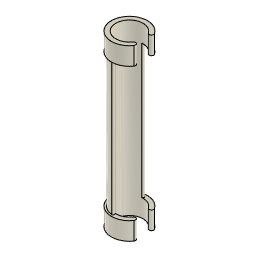
LaptopArmHolder v2 (Autodesk Fusion 360 design; units mm, degrees)
Autodesk Fusion 360 part; units mm, degrees
sketch "Sketch1" plane through (0, 0, 0) normal (0, 0, 1) x (1, 0, 0)
  circle A0 centre (14.5763, 12.4188) radius 15.25
  circle A1 centre (14.5763, 12.4188) radius 18.25
  circle A2 centre (14.5763, 12.4188) radius 20.25
  line L0 (14.5763, 32.6688) -> (14.5763, -7.8312)
  dimension "d1" = 30.5
  dimension "d2" = 36.5
  dimension "d6" = 40.5
  constraint concentric A0 A1
  constraint concentric A1 A2
  constraint coincident A2 L0.start
  constraint coincident A2 L0.end
  constraint vertical L0
  measures "d1" diameter of A0
  measures "d2" diameter of A1
  measures "d6" diameter of A2
extrude "Extrude1" add sketch "Sketch1" along normal blind 150 contours A0 A1 L0 picked at (13.6696, 29.6009)
sketch "Sketch2" plane through (0, 0, 150) normal (0, 0, 1) x (-1, 0, 0)
  arc A0 (-14.5763, -30.6688) -> (-14.5763, 5.8312) centre (-14.5763, -12.4188) ccw
  arc A1 (-14.5763, -27.6688) -> (-14.5763, 2.8312) centre (-14.5763, -12.4188) ccw
  circle A2 centre (-14.5763, -12.4188) radius 15.25
  circle A3 centre (-14.5763, -12.4188) radius 20.25
  line L0 (-14.5763, -32.6688) -> (-14.5763, 7.8312)
  line L1 (-14.5763, -27.6688) -> (-14.5763, -30.6688)
  line L2 (-14.5763, 5.8312) -> (-14.5763, 2.8312)
  line L3 (-14.5763, -27.6688) -> (-14.5763, -12.4188)
  line L4 (-14.5763, 2.8312) -> (-14.5763, -12.4188)
  line L5 (-14.5763, -4.7938) -> (-33.3359, -4.7938)
  line L6 (-14.5763, -20.0438) -> (-33.3359, -20.0438)
  dimension "d5" = 40.5
  constraint concentric A0 A2
  constraint concentric A2 A3
  constraint coincident A3 L0.start
  constraint coincident A3 L0.end
  constraint coincident A1.start L1.start
  constraint coincident A0.centre A1.centre
  constraint parallel L0 L3
  constraint coincident A1.end L2.end
  constraint midpoint L4 L5.start
  constraint coincident A3 L5.end
  constraint perpendicular L4 L5
  constraint midpoint L3 L6.start
  constraint coincident A3 L6.end
  constraint perpendicular L3 L6
  measures "d5" diameter of A3
extrude "Extrude2" add sketch "Sketch2" along normal blind 20 contours A0 A1 A2 L0 L1 L2 | A0 A3 L0 | A2 A3 L0 L1 L6 | A2 A3 L0 L2 L5
sketch "Sketch3" plane through (0, 0, 0) normal (0, 0, 1) x (1, 0, 0)
  circle A0 centre (14.5763, 12.4188) radius 15.25
  line L0 (14.5763, 32.6688) -> (14.5763, -7.8312)
  line L1 (14.5763, -2.8312) -> (14.5763, 12.4188)
  line L2 (14.5763, 12.4188) -> (14.5763, 27.6688)
  circle A1 centre (14.5763, 12.4188) radius 20.25
  line L3 (14.5763, 20.0438) -> (33.3359, 20.0438)
  line L4 (14.5763, 4.7938) -> (33.3359, 4.7938)
  point P0 (14.5763, 12.4188)
  constraint coincident A0 L1.start
  constraint coincident L0 L1.start
  constraint coincident P0 A0.centre
  constraint coincident L0 L2.end
  constraint coincident A0 L2.end
  constraint midpoint L2 L3.start
  constraint coincident A1 L3.end
  constraint perpendicular L2 L3
  constraint midpoint L1 L4.start
  constraint coincident A1 L4.end
  constraint perpendicular L0 L4
extrude "Extrude3" add sketch "Sketch1" sketch "Sketch3" against normal blind 20 contours A0 A1 L0 picked at (13.6696, 29.6009) of sketch 2 contours A0 L0 A1 L3 | A0 L0 A1 | A0 L0 A1 L4
fillet "Fillet1" radius 2.5 2 edges at (27.7832, 20.0438, 160) (33.3359, 20.0438, 160)
fillet "Fillet2" radius 2.5 6 edges at (27.7832, 4.7938, 160) (33.3359, 4.7938, 160) (27.7832, 4.7938, -10) (33.3359, 4.7938, -10) (33.3359, 20.0438, -10) (27.7832, 20.0438, -10)
fillet "Fillet3" radius 1.5 4 edges at (14.5763, -5.8312, 75) (14.5763, -2.8312, 75) (14.5763, 30.6688, 75) (14.5763, 27.6688, 75)
